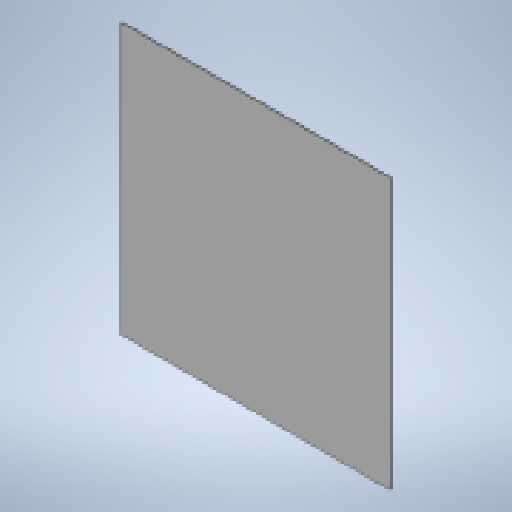
# Autodesk Inventor part: GBK 1111 shield 1
Saved by Autodesk Inventor 2026 (Build 300175000, 175)
## iProperties
Created: 2026-04-17
Part Number: GBK 1111 shield 1
Material: Steel
Document SubType Name: Sheet Metal
Designer: admin
Density: 7.85 g/cm^3
Sheet Metal Rule: По умолчанию_мм
Appearance: Default
Mass: 69243.3 g
Surface Area: 44341.6 cm^2
Volume: 8820.8 cm^3
Flat Pattern Width: 148 cm
Flat Pattern Length: 149 cm
Flat Pattern Area: 22052 cm^2
Sheet Metal Width: 1480,000 мм
Sheet Metal Length: 1490,000 мм
Sheet Metal Area: 2205200,000 мм^2
Stock Number: 1115
Author: admin
Autodesk Inventor part; units mm, degrees
ref_plane "YZ Plane" through (0, 0, 0) normal (1, 0, 0) x (0, 1, 0)
ref_plane "XZ Plane" through (0, 0, 0) normal (0, 1, 0) x (-1, 0, 0)
ref_plane "XY Plane" through (0, 0, 0) normal (0, 0, 1) x (1, 0, 0)
sketch "Sketch1" plane through (0, 0, 0) normal (0, 0, 1) x (1, 0, 0)
  line L0 (740, -745) -> (-740, -745)
  line L1 (-740, -745) -> (-740, 745)
  line L2 (-740, 745) -> (740, 745)
  line L3 (740, 745) -> (740, -745)
  line L4 (740, -745) -> (-740, 745) construction
  line L5 (-740, -745) -> (740, 745) construction
  point P0 (0, 0)
  dimension "d0" = 1480
  dimension "d1" = 1490
  measures "d0" distance of L1.end L2.end
  measures "d1" distance of L0.end L1.end
extrude "Plate1" add sketch "Sketch1" along normal blind 4
sketch "Sketch3" plane through (0, 0, 0) normal (0, 0, -1) x (-1, 0, 0)
  line L0 (669.8628, -494.5) -> (669.8628, -591.5)
  line L1 (669.8628, -591.5) -> (665.8638, -591.5)
  line L2 (169.7342, -494.5) -> (169.7342, -591.5)
  line L3 (169.7342, -591.5) -> (165.7352, -591.5)
  line L4 (-330.3944, -494.5) -> (-330.3944, -591.5)
  line L5 (-330.3944, -591.5) -> (-334.3934, -591.5)
  ellipse E0 centre (-330.3944, 743.5) end of major axis (-330.3944, 773.5) minor radius 0.6803 (-330.3944, 713.5) -> (-330.3944, 773.5) ccw
  line L6 (-330.3944, 713.5) -> (-334.3934, 713.5)
  ellipse E1 centre (169.7342, 743.5) end of major axis (169.7342, 773.5) minor radius 0.6803 (169.7342, 713.5) -> (169.7342, 773.5) ccw
  line L7 (169.7342, 713.5) -> (165.7352, 713.5)
  ellipse E2 centre (669.8628, 743.5) end of major axis (669.8628, 773.5) minor radius 0.6803 (669.8628, 713.5) -> (669.8628, 773.5) ccw
  line L8 (669.8628, 713.5) -> (665.8638, 713.5)
  line L9 (710, -491) -> (770, -491)
  line L10 (710, -491) -> (710, -487)
  line L11 (710, 5.6667) -> (770, 5.6667)
  line L12 (710, 5.6667) -> (710, 9.6667)
  line L13 (710, 502.3333) -> (770, 502.3333)
  line L14 (710, 502.3333) -> (710, 506.3333)
  line L15 (-738.6395, 502.3333) -> (-680, 502.3333)
  line L16 (-680, 502.3333) -> (-680, 506.3333)
  line L17 (-738.6395, 5.6667) -> (-680, 5.6667)
  line L18 (-680, 5.6667) -> (-680, 9.6667)
  line L19 (-738.6395, -491) -> (-680, -491)
  line L20 (-680, -491) -> (-680, -487)
  line L21 (488.1353, -557.3462) -> (488.1353, -1055.4823) construction
  line L22 (488.1353, -1055.4823) -> (448.5081, -1055.4823) construction
  line L23 (448.5081, -1055.4823) -> (448.5081, -557.3462) construction
  line L24 (448.5081, -557.3462) -> (488.1353, -557.3462) construction
  constraints: 42 end point, 12 horizontal, 9 vertical, 53 other
mark "Mark2"
equation "\"d0\" = Лист_ширина"
equation "\"d1\" = 0.5 * Лист_длина"
equation "\"d2\" = Thickness"
equation "\"BendRadius\" = Thickness"
equation "\"BendReliefWidth\" = Thickness"
equation "\"BendReliefDepth\" = 0.5 * Thickness"
equation "\"CornerReliefSize\" = 4 * Thickness"
equation "\"MinimumRemnant\" = 2 * Thickness"
equation "\"TransitionRadius\" = BendRadius"
equation "\"JacobiRadiusSize\" = BendRadius"
equation "\"GapSize\" = Thickness"
equation "\"Лист_ширина\" = 1480"
equation "\"Лист_длина\" = 2980"
equation "\"Thickness\" = 4"
body "Solid1"
